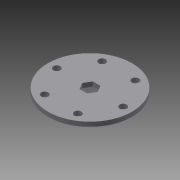
# Autodesk Inventor part: Pneumatic Hub
Saved by Autodesk Inventor 2013 (Build 170138000, 138)
## iProperties
Created: 2013-01-19
Part Number: Pneumatic Hub
Material: Generic
Document SubType Name: Modeling
Designer: actoennies
Density: 1 g/cm^3
Author: actoennies
Autodesk Inventor part; units mm, degrees
ref_plane "YZ Plane" through (0, 0, 0) normal (1, 0, 0) x (0, 1, 0)
ref_plane "XZ Plane" through (0, 0, 0) normal (0, 1, 0) x (-1, 0, 0)
ref_plane "XY Plane" through (0, 0, 0) normal (0, 0, 1) x (1, 0, 0)
sketch "Sketch1" plane through (0, 0, 0) normal (0, 1, 0) x (-1, 0, 0)
  circle A0 centre (-23.8125, 0) radius 2.54
  line L0 (2.7496, 4.7625) -> (5.4993, 0)
  line L1 (5.4993, 0) -> (2.7496, -4.7625)
  line L2 (2.7496, -4.7625) -> (-2.7496, -4.7625)
  line L3 (-2.7496, -4.7625) -> (-5.4993, 0)
  line L4 (-5.4993, 0) -> (-2.7496, 4.7625)
  line L5 (-2.7496, 4.7625) -> (2.7496, 4.7625)
  circle A1 centre (-11.9063, 20.6222) radius 2.54
  circle A2 centre (11.9062, 20.6222) radius 2.54
  circle A3 centre (23.8125, 0) radius 2.54
  circle A4 centre (-11.9063, -20.6222) radius 2.54
  circle A5 centre (11.9062, -20.6222) radius 2.54
  circle A6 centre (0, 0) radius 30.1625
  dimension "d0" = 5.08
  dimension "d6" = 5.08
  dimension "d8" = 5.08
  dimension "d10" = 5.08
  dimension "d11" = 60.325
  dimension "d12" = 9.525
  constraints: 12 end point, 7 centre point, 1 coincident, 15 other
  measures "d0" diameter of A0
  measures "d6" diameter of A1
  measures "d8" diameter of A3
  measures "d10" diameter of A4
  measures "d11" diameter of A6
  measures "d12" distance between parallel lines of L2 L5
extrude "Extrusion1" add sketch "Sketch1" along normal blind 3.175
body "Solid1"
